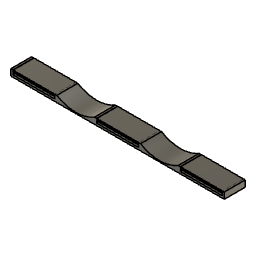
ACUTE_Millistykki v1 (Autodesk Fusion 360 design; units mm, degrees)
Autodesk Fusion 360 part; units mm, degrees
sketch "Sketch1" plane through (0, 0, 0) normal (0, 1, 0) x (1, 0, 0)
  line L0 (0, 0) -> (20, 0)
  line L1 (20, 0) -> (20, -1)
  line L2 (19.9, -1) -> (0, -1)
  line L3 (0, -1) -> (0, 0)
  line L4 (0, -1) -> (-1, -1) construction
  line L5 (-1, -1) -> (-1, -2) construction
  line L6 (-1, -2) -> (0, -2) construction
  line L7 (0, -2) -> (0, -1) construction
  line L8 (20, 0) -> (21, 0) construction
  line L9 (21, 0) -> (21, 1) construction
  line L10 (21, 1) -> (20, 1) construction
  line L11 (20, 1) -> (20, 0) construction
  line L12 (21, -2) -> (21, 1)
  line L13 (21, 1) -> (-1, 1)
  line L14 (-1, 1) -> (-1, -2)
  line L15 (20, -1) -> (20, -1.5)
  line L16 (19.9, -1.5) -> (0, -1.5)
  line L17 (0, -1.5) -> (0, -2)
  line L18 (0.1, -2) -> (0.1, -1.6)
  line L19 (0.1, -1.6) -> (20, -1.6)
  line L20 (20, -1.6) -> (19.9, -1.6) construction
  line L21 (19.9, -1.5) -> (19.9, -1)
  line L22 (-1, -2) -> (0, -2)
  line L23 (0.1, -2) -> (21, -2)
  line L24 (0, -1.5) -> (0, -1)
  line L25 (20, -1.5) -> (20, -1.6)
  dimension "d1" = 20
  dimension "d2" = 1
  dimension "d3" = 1
  dimension "d4" = 1
  dimension "d5" = 1
  dimension "d6" = 1
  dimension "d7" = 0.5
  dimension "d8" = 0.1
  dimension "d9" = 0.4
  dimension "d10" = 0.1
  constraint horizontal L0
  constraint vertical L1
  constraint horizontal L2
  constraint vertical L3
  constraint coincident L0.start L3.end
  constraint horizontal L4
  constraint vertical L5
  constraint horizontal L6
  constraint vertical L7
  constraint horizontal L8
  constraint vertical L9
  constraint horizontal L10
  constraint vertical L11
  constraint horizontal L22
  constraint vertical L12
  constraint horizontal L13
  constraint vertical L14
  constraint perpendicular L2 L15
  constraint midpoint L7 L16.end
  constraint perpendicular L16 L18
  constraint perpendicular L15 L19
  constraint parallel L19 L20
  constraint perpendicular L2 L21
  constraint collinear L22 L23
  constraint perpendicular L19 L25
  measures "d1" distance of L0.start L0.end
  measures "d2" distance of L0.start L2.end
  measures "d3" distance of L2.end L4.end
  measures "d4" distance of L2.end L6.end
  measures "d5" distance of L0.end L8.end
  measures "d6" distance of L0.end L10.end
  measures "d7" distance of L1.end L15.end
  measures "d8" distance of L6.end L18.start
  measures "d9" distance of L18.start L18.end
  measures "d10" distance of L19.end L20.end
extrude "Extrude1" add sketch "Sketch1" along normal blind 10 makes body 1
pattern_linear "R-Pattern1" count 3 spacing 40 along (1, 0, 0) of bodies 1 makes body 2 at (53.6667, 3.3333, -1) makes body 3 at (93.6667, 3.3333, -1)
sketch "Sketch2" plane through (0, 0, -1) normal (0, 0, -1) x (1, 0, 0)
  line L0 (21, 0) -> (-1, 0)
  line L1 (-1, 0) -> (-1, -10)
  line L2 (-1, -10) -> (21, -10)
  line L3 (21, -10) -> (21, 0)
  line L4 (21, 0) -> (39, 0)
  line L5 (39, 0) -> (39, -10)
  line L6 (39, -10) -> (21, -10)
  line L7 (21, -10) -> (21, 0)
  line L8 (61, 0) -> (79, 0)
  line L9 (79, 0) -> (79, -10)
  line L10 (79, -10) -> (61, -10)
  line L11 (61, -10) -> (61, 0)
  point P0 (39, -10)
  point P1 (61, 0)
  point P2 (79, -10)
  constraint horizontal L4
  constraint vertical L5
  constraint horizontal L6
  constraint vertical L7
  constraint coincident P0 L5.end
  constraint coincident L0.start L3.end
  constraint horizontal L8
  constraint vertical L9
  constraint horizontal L10
  constraint vertical L11
  constraint coincident P2 L9.end
  constraint coincident P1 L8.start
extrude "Extrude2" add sketch "Sketch2" against normal blind 0.5 contours L3 L4 L5 L6 L7 | L8 L9 L10 L11 bodies 1 2 3
fillet "Fillet1" radius 17.5 4 edges at (21, 5, -0.5) (61, 5, -0.5) (39, 5, -0.5) (79, 5, -0.5) on bodies 1
